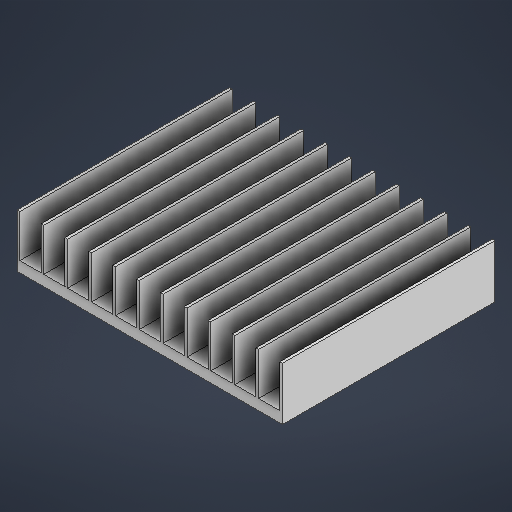
# Autodesk Inventor part: Heatsink_and_Amplifier
Saved by Autodesk Inventor 2026.2 (Build 302298010, 298A)
## iProperties
Created: 2026-09-21
Part Number: Heatsink_and_Amplifier
Material: Generic
Document SubType Name: Modeling
Designer: aiden
Density: 1 g/cm^3
Appearance: Default
Author: aiden
Autodesk Inventor part; units mm, degrees
ref_plane "YZ Plane" through (0, 0, 0) normal (1, 0, 0) x (0, 1, 0)
ref_plane "XZ Plane" through (0, 0, 0) normal (0, 1, 0) x (-1, 0, 0)
ref_plane "XY Plane" through (0, 0, 0) normal (0, 0, 1) x (1, 0, 0)
sketch "Sketch1" plane through (0, 0, 0) normal (0, 1, 0) x (-1, 0, 0)
  line L0 (-63.5, -50.8) -> (63.5, -50.8)
  line L1 (63.5, -50.8) -> (63.5, 50.8)
  line L2 (63.5, 50.8) -> (-63.5, 50.8)
  line L3 (-63.5, 50.8) -> (-63.5, -50.8)
  line L4 (-63.5, -50.8) -> (63.5, 50.8) construction
  line L5 (63.5, -50.8) -> (-63.5, 50.8) construction
  point P0 (0, 0)
  dimension "d0" = 127
  dimension "d1" = 101.6
  constraints: 12 end point, 2 midpoint, 2 parallel, 1 horizontal, 1 perpendicular
  measures "d0" distance of L2.end L1.end
  measures "d1" distance of L1.end L0.end
extrude "Extrusion1" add sketch "Sketch1" along normal blind 25.4
sketch "Sketch2" plane through (-63.5, 0, 50.8) normal (0, 0, 1) x (1, 0, 0)
  line L0 (0, 0) -> (127, 0) projected
  line L1 (0, 0) -> (0, 5.08)
  line L2 (0, 25.4) -> (127, 25.4) projected
  line L3 (0, 5.08) -> (127, 5.08) construction
  line L4 (127, 0) -> (0, 0)
  line L5 (0, 5.08) -> (0, 25.4)
  line L6 (0, 25.4) -> (1.27, 25.4)
  line L7 (1.27, 25.4) -> (1.27, 5.08)
  line L8 (1.27, 5.08) -> (0, 5.08)
  line L9 (127, 0) -> (127, 25.4) projected
  line L10 (127, 25.4) -> (127, 0)
  line L11 (11.43, 5.08) -> (11.43, 25.4)
  line L12 (11.43, 25.4) -> (12.7, 25.4)
  line L13 (12.7, 25.4) -> (12.7, 5.08)
  line L14 (12.7, 5.08) -> (11.43, 5.08)
  line L15 (22.86, 5.08) -> (22.86, 25.4)
  line L16 (22.86, 25.4) -> (24.13, 25.4)
  line L17 (24.13, 25.4) -> (24.13, 5.08)
  line L18 (24.13, 5.08) -> (22.86, 5.08)
  line L19 (34.29, 5.08) -> (34.29, 25.4)
  line L20 (34.29, 25.4) -> (35.56, 25.4)
  line L21 (35.56, 25.4) -> (35.56, 5.08)
  line L22 (35.56, 5.08) -> (34.29, 5.08)
  line L23 (45.72, 5.08) -> (45.72, 25.4)
  line L24 (45.72, 25.4) -> (46.99, 25.4)
  line L25 (46.99, 25.4) -> (46.99, 5.08)
  line L26 (46.99, 5.08) -> (45.72, 5.08)
  line L27 (57.15, 5.08) -> (57.15, 25.4)
  line L28 (57.15, 25.4) -> (58.42, 25.4)
  line L29 (58.42, 25.4) -> (58.42, 5.08)
  line L30 (58.42, 5.08) -> (57.15, 5.08)
  line L31 (68.58, 5.08) -> (68.58, 25.4)
  line L32 (68.58, 25.4) -> (69.85, 25.4)
  line L33 (69.85, 25.4) -> (69.85, 5.08)
  line L34 (69.85, 5.08) -> (68.58, 5.08)
  line L35 (80.01, 5.08) -> (80.01, 25.4)
  line L36 (80.01, 25.4) -> (81.28, 25.4)
  line L37 (81.28, 25.4) -> (81.28, 5.08)
  line L38 (81.28, 5.08) -> (80.01, 5.08)
  line L39 (91.44, 5.08) -> (91.44, 25.4)
  line L40 (91.44, 25.4) -> (92.71, 25.4)
  line L41 (92.71, 25.4) -> (92.71, 5.08)
  line L42 (92.71, 5.08) -> (91.44, 5.08)
  line L43 (102.87, 5.08) -> (102.87, 25.4)
  line L44 (102.87, 25.4) -> (104.14, 25.4)
  line L45 (104.14, 25.4) -> (104.14, 5.08)
  line L46 (104.14, 5.08) -> (102.87, 5.08)
  line L47 (114.3, 5.08) -> (114.3, 25.4)
  line L48 (114.3, 25.4) -> (115.57, 25.4)
  line L49 (115.57, 25.4) -> (115.57, 5.08)
  line L50 (115.57, 5.08) -> (114.3, 5.08)
  line L51 (125.73, 5.08) -> (125.73, 25.4)
  line L52 (125.73, 25.4) -> (127, 25.4)
  line L53 (127, 25.4) -> (127, 5.08)
  line L54 (127, 5.08) -> (125.73, 5.08)
  line L55 (0, 25.4) -> (127, 25.4)
  line L56 (127, 25.4) -> (127, 5.08)
  line L57 (127, 5.08) -> (0, 5.08)
  line L58 (0, 5.08) -> (0, 25.4)
  point P0 (0.635, 25.4)
  point P1 (12.065, 25.4)
  point P2 (23.495, 25.4)
  point P3 (34.925, 25.4)
  point P4 (46.355, 25.4)
  point P5 (57.785, 25.4)
  point P6 (69.215, 25.4)
  point P7 (80.645, 25.4)
  point P8 (92.075, 25.4)
  point P9 (103.505, 25.4)
  point P10 (114.935, 25.4)
  point P11 (126.365, 25.4)
  point P12 (126.365, 25.4)
  point P13 (12.7, 5.08)
  point P14 (12.7, 25.4)
  point P15 (1.27, 5.08)
  point P16 (1.27, 25.4)
  dimension "d4" = 5.08
  dimension "d5" = 1.27
  dimension "d36" = 11.43
  dimension "d41" = 0.635
  constraints: 110 end point, 4 perpendicular, 3 horizontal, 2 collinear, 2 midpoint, 2 point on line, 1 parallel, 1 vertical, 103 other
  measures "d4" distance of L0.start L1.end
  measures "d5" distance between parallel lines of L5 L7
  measures "d36" distance of L1.end L11.start
  measures "d41" distance of L9.end point (126.365, 25.4)
extrude "Extrusion2" cut sketch "Sketch2" against normal blind 122.2375 contours L7 L2 L11 L57 | L57 L49 L2 L51 | L13 L2 L15 L57 | L57 L45 L2 L47 | L17 L2 L19 L57 | L57 L41 L2 L43 | L21 L2 L23 L57 | L57 L37 L2 L39 | L25 L2 L27 L57 | L57 L33 L2 L35 | L29 L2 L31 L57
body "Solid1"
